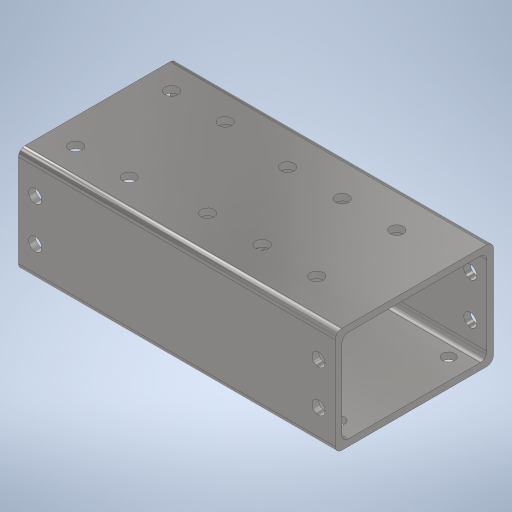
# Autodesk Inventor part: 3x6_Bar
Saved by Autodesk Inventor 2023 (Build 270158000, 158)
## iProperties
Created: 2025-04-19
Part Number: 3x6_Bar
Material: Steel, Mild
Document SubType Name: Modeling
Designer: plebbb
Density: 7.85 g/cm^3
Appearance: Semi-Polished
Author: plebbb
Autodesk Inventor part; units mm, degrees
ref_plane "YZ Plane" through (0, 0, 0) normal (1, 0, 0) x (0, 1, 0)
ref_plane "XZ Plane" through (0, 0, 0) normal (0, 1, 0) x (-1, 0, 0)
sketch "Sketch1" plane through (0, 0, 0) normal (1, 0, 0) x (0, 1, 0)
  line L0 (0, 0) -> (50.8, 0)
  line L1 (50.8, 0) -> (50.8, -76.2)
  line L2 (50.8, -76.2) -> (0, -76.2)
  line L3 (0, -76.2) -> (0, 0)
  dimension "d0" = 76.2
  dimension "d1" = 50.8
  constraints: 8 end point, 2 parallel, 1 horizontal, 1 perpendicular
  measures "d0" distance of L0.end L1.end
  measures "d1" distance of L1.end L2.end
extrude "Extrusion1" add sketch "Sketch1" along normal blind 152.4
shell "Shell1" thickness 3.175 removed faces 2 at (0, 33.8667, -50.8) at (152.4, 33.8667, -50.8)
fillet "Fillet1" radius 3.175 8 edges at (76.2, 50.8, -76.2) (76.2, 50.8, 0) (76.2, 0, -76.2) (76.2, 0, 0) (76.2, 3.175, -3.175) (76.2, 3.175, -73.025) (76.2, 47.625, -3.175) (76.2, 47.625, -73.025)
sketch "Sketch2" plane through (0, 0, -73.025) normal (0, -1, 0) x (1, 0, 0)
  circle A0 centre (142.4, 61.425) radius 3
  line L0 (142.4, 61.425) -> (102.4, 61.425) construction
  line L1 (102.4, 61.425) -> (102.4, 8.425) construction
  line L2 (102.4, 8.425) -> (142.4, 8.425) construction
  line L3 (142.4, 8.425) -> (142.4, 61.425) construction
  line L4 (152.4, 69.85) -> (152.4, 0) construction
  line L5 (152.4, 66.675) -> (152.4, 3.175) construction
  line L6 (152.4, 34.925) -> (142.4, 34.925) construction
  circle A1 centre (142.4, 8.425) radius 3
  circle A2 centre (102.4, 61.425) radius 3
  circle A3 centre (102.4, 8.425) radius 3
  point P0 (0, 73.025)
  dimension "d6" = 6
  dimension "d7" = 53
  dimension "d8" = 40
  dimension "d9" = 10
  constraints: 10 end point, 4 centre point, 3 coincident, 3 equal radius, 2 midpoint, 2 parallel, 2 perpendicular, 1 horizontal
  measures "d6" diameter of A0
  measures "d7" distance of L2.end L0.start
  measures "d8" distance of L1.end L2.end
  measures "d9" distance of L6.start L6.end
ref_plane "Work Plane1" through (76.2, 0, 0) normal (1, 0, 0) x (0, 0, -1)
extrude "Extrusion2" cut sketch "Sketch2" against normal up to surface (3.175 mm away)
mirror "Mirror1" about plane through (76.2, 0, 0) normal (1, 0, 0) of "Extrusion2"
sketch "Sketch3" plane through (0, 50.8, -3.175) normal (0, 1, 0) x (1, 0, 0)
  line L0 (12.5, 58.025) -> (38.3, 58.025) construction
  line L1 (38.3, 58.025) -> (38.3, 11.825) construction
  line L2 (38.3, 11.825) -> (12.5, 11.825) construction
  line L3 (12.5, 11.825) -> (12.5, 58.025) construction
  circle A0 centre (12.5, 58.025) radius 3.175
  circle A1 centre (38.3, 58.025) radius 3.175
  circle A2 centre (12.5, 11.825) radius 3.175
  circle A3 centre (38.3, 11.825) radius 3.175
  line L4 (0, -3.175) -> (50.8, -3.175) construction
  line L5 (50.8, -3.175) -> (50.8, 73.025) construction
  line L6 (50.8, 73.025) -> (0, 73.025) construction
  line L7 (0, 73.025) -> (0, -3.175) construction
  line L8 (38.3, 34.925) -> (50.8, 34.925) construction
  line L9 (25.4, 58.025) -> (25.4, 73.025) construction
  dimension "d12" = 6.35
  dimension "d13" = 50.8
  dimension "d14" = 76.2
  dimension "d16" = 15
  dimension "d17" = 12.5
  constraints: 20 end point, 4 centre point, 4 coincident, 4 midpoint, 4 parallel, 4 perpendicular, 3 equal radius, 2 horizontal, 1 horizontal alignment, 1 vertical alignment
  measures "d12" diameter of A0
  measures "d13" distance of L5.end L6.end
  measures "d14" distance of L4.end L5.end
  measures "d16" distance of L9.start L9.end
  measures "d17" distance of L8.start L8.end
extrude "Extrusion3" cut sketch "Sketch3" against normal up to surface (3.175 mm away)
sketch "Sketch4" plane through (0, 50.8, -3.175) normal (0, 1, 0) x (1, 0, 0)
  line L0 (50.8, -3.175) -> (152.4, -3.175) construction
  line L1 (152.4, -3.175) -> (152.4, 73.025) construction
  line L2 (152.4, 73.025) -> (50.8, 73.025) construction
  line L3 (50.8, 73.025) -> (50.8, -3.175) construction
  line L4 (152.4, 66.675) -> (50.8, 66.675) construction
  line L5 (50.8, 66.675) -> (50.8, 3.175) construction
  line L6 (50.8, 3.175) -> (152.4, 3.175) construction
  line L7 (152.4, 3.175) -> (152.4, 66.675) construction
  line L8 (101.6, 66.675) -> (101.6, 73.025) construction
  line L9 (101.6, 3.175) -> (101.6, -3.175) construction
  line L10 (72.15, 54.175) -> (124.7, 54.175) construction
  line L11 (124.7, 54.175) -> (124.7, 15.675) construction
  line L12 (124.7, 15.675) -> (72.15, 15.675) construction
  line L13 (72.15, 15.675) -> (72.15, 54.175) construction
  circle A0 centre (72.15, 54.175) radius 3.175
  circle A1 centre (72.15, 15.675) radius 3.175
  circle A2 centre (98.425, 15.675) radius 3.175
  circle A3 centre (98.425, 54.175) radius 3.175
  circle A4 centre (124.7, 54.175) radius 3.175
  circle A5 centre (124.7, 15.675) radius 3.175
  line L14 (57.15, 66.675) -> (57.15, 3.175) construction
  line L15 (57.15, 34.925) -> (72.15, 34.925) construction
  line L16 (124.7, 34.925) -> (139.7, 34.925) construction
  line L17 (139.7, 3.175) -> (139.7, 66.675) construction
  point P0 (0, -3.175)
  dimension "d20" = 101.6
  dimension "d21" = 76.2
  dimension "d22" = 50.8
  dimension "d23" = 63.5
  dimension "d24" = 6.35
  dimension "d25" = 6.35
  dimension "d26" = 12.5
  dimension "d27" = 15
  dimension "d31" = 88.9
  constraints: 36 end point, 10 midpoint, 6 centre point, 6 parallel, 6 point on line, 5 equal radius, 5 perpendicular, 4 coincident, 4 horizontal, 2 collinear, 1 horizontal alignment, 1 vertical
  measures "d20" distance of L1.end L2.end
  measures "d21" distance of L0.end L1.end
  measures "d22" distance of point (0, -3.175) L0.start
  measures "d23" distance between parallel lines of L6 L4
  measures "d24" diameter of A0
  measures "d25" distance between parallel lines of L3 L14
  measures "d26" distance between parallel lines of L4 L10
  measures "d27" distance of L15.start L15.end
  measures "d31" distance from line of L17 L0.start
extrude "Extrusion4" cut sketch "Sketch4" against normal up to surface (3.175 mm away)
sketch "Sketch5" plane through (0, 3.175, -76.2) normal (0, 0, -1) x (-1, 0, 0)
  circle A0 centre (-8, 32.225) radius 3.175
  circle A1 centre (-8, 12.225) radius 3.175
  line L0 (0, -3.175) -> (-16, -3.175) construction
  line L1 (-16, -3.175) -> (-16, 47.625) construction
  line L2 (-16, 47.625) -> (0, 47.625) construction
  line L3 (0, 47.625) -> (0, -3.175) construction
  line L4 (-8, 32.225) -> (-8, 47.625) construction
  line L5 (-8, 12.225) -> (-8, -3.175) construction
  dimension "d32" = 50.8
  dimension "d33" = 16
  dimension "d34" = 6.35
  dimension "d35" = 20
  constraints: 12 end point, 3 perpendicular, 2 centre point, 2 midpoint, 2 parallel, 1 collinear, 1 equal radius, 1 horizontal
  measures "d32" distance of L2.end L0.start
  measures "d33" distance of L1.end L2.end
  measures "d34" diameter of A0
  measures "d35" distance of L5.start L4.start
extrude "Extrusion5" cut sketch "Sketch5" against normal through all
mirror "Mirror2" about plane through (76.2, 0, 0) normal (1, 0, 0) of "Extrusion5"
equation "\"BendRadius\" = Thickness"
equation "\"BendReliefWidth\" = Thickness"
equation "\"BendReliefDepth\" = 0.5 * Thickness"
equation "\"CornerReliefSize\" = 4 * Thickness"
equation "\"MinimumRemnant\" = 2 * Thickness"
equation "\"TransitionRadius\" = BendRadius"
equation "\"JacobiRadiusSize\" = BendRadius"
equation "\"GapSize\" = Thickness"
equation "\"Thickness\" = 3.048"
body "Solid1"
